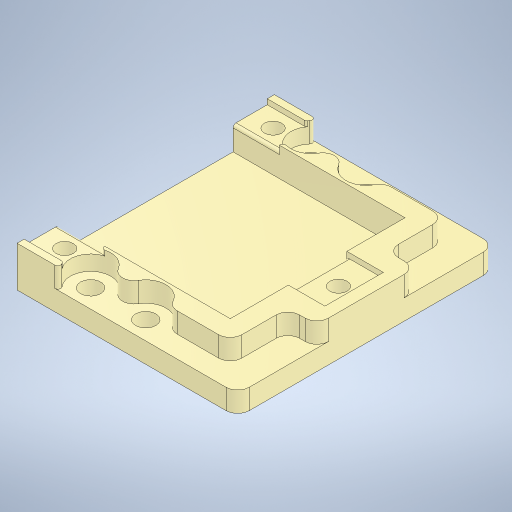
# Autodesk Inventor part: Servo Support
Saved by Autodesk Inventor 2023.4 (Build 274418000, 418)
## iProperties
Created: 2024-01-22
Part Number: Servo Support
Material: Nylon 6/6
Document SubType Name: Modeling
Designer: Nathan Cai
Density: 1.13 g/cm^3
Appearance: Nylon 6
Mass: 6.26234 g
Surface Area: 50.527 cm^2
Volume: 5.5419 cm^3
Author: Nathan Cai
Autodesk Inventor part; units mm, degrees
ref_plane "YZ Plane" through (0, 0, 0) normal (1, 0, 0) x (0, 1, 0)
ref_plane "XZ Plane" through (0, 0, 0) normal (0, 1, 0) x (-1, 0, 0)
ref_plane "XY Plane" through (0, 0, 0) normal (0, 0, 1) x (1, 0, 0)
sketch "Sketch8" plane through (0, 0, 0) normal (0, 1, 0) x (-1, 0, 0)
  line L0 (-14.8, 15) -> (14.8, 15)
  line L1 (14.8, 15) -> (14.8, -15)
  line L2 (14.8, -15) -> (-14.8, -15)
  line L3 (-14.8, -15) -> (-14.8, 15)
  line L4 (-14.8, 15) -> (14.8, -15) construction
  line L5 (14.8, 15) -> (-14.8, -15) construction
  line L6 (14.8, 0) -> (-14.8, 0) construction
  line L7 (14.8, 21) -> (6.8, 21)
  line L8 (6.8, 21) -> (6.8, -21)
  line L9 (6.8, -21) -> (14.8, -21)
  line L10 (14.8, -21) -> (14.8, 21)
  line L11 (14.8, 21) -> (6.8, -21) construction
  line L12 (6.8, 21) -> (14.8, -21) construction
  line L13 (10.8, 21) -> (10.8, -21) construction
  circle A0 centre (10.8, 18) radius 1.5
  circle A1 centre (10.8, -18) radius 1.5
  line L14 (-21.2, 5.05) -> (-14.8, 5.05)
  line L15 (-14.8, 5.05) -> (-14.8, -5.05)
  line L16 (-14.8, -5.05) -> (-21.2, -5.05)
  line L17 (-21.2, -5.05) -> (-21.2, 5.05)
  line L18 (-21.2, 5.05) -> (-14.8, -5.05) construction
  line L19 (-14.8, 5.05) -> (-21.2, -5.05) construction
  circle A2 centre (-18.5, 0) radius 1.5
  line L20 (24.325, 14.4) -> (14.8, 14.4)
  line L21 (14.8, 14.4) -> (14.8, 2.4)
  line L22 (14.8, 2.4) -> (24.325, 2.4)
  line L23 (24.325, 2.4) -> (24.325, 14.4)
  line L24 (24.325, 14.4) -> (14.8, 2.4) construction
  line L25 (14.8, 14.4) -> (24.325, 2.4) construction
  line L26 (-23.3, 22.225) -> (14.8, 22.225)
  line L27 (14.8, 22.225) -> (14.8, -22.225)
  line L28 (14.8, -22.225) -> (-23.3, -22.225)
  line L29 (-23.3, -22.225) -> (-23.3, 22.225)
  line L30 (-23.3, 22.225) -> (14.8, -22.225) construction
  line L31 (14.8, 22.225) -> (-23.3, -22.225) construction
  point P0 (0, 0)
  point P1 (10.8, 0)
  point P2 (-18, 0)
  point P3 (19.5625, 8.4)
  point P4 (-4.25, 0)
  point P5 (14.8, 21)
  point P6 (-14.8, 5.05)
  point P7 (6.8, -15)
  point P8 (14.8, 15)
  point P9 (6.8, 15)
  dimension "d120" = 29.6
  dimension "d121" = 30
  dimension "d122" = 8
  dimension "d123" = 42
  dimension "d124" = 3
  dimension "d126" = 36
  dimension "d127" = 10.1
  dimension "d128" = 36
  dimension "d129" = 3
  dimension "d130" = 29.3
  dimension "d131" = 9.6
  dimension "d132" = 12
  dimension "d133" = 9.525
  dimension "d134" = 44.45
  dimension "d135" = 38.1
  constraints: 64 end point, 14 midpoint, 10 parallel, 9 point on line, 5 horizontal, 5 perpendicular, 3 centre point, 1 symmetric about line, 1 other
  measures "d120" distance of L1.end L2.end
  measures "d121" distance of L0.end L1.end
  measures "d122" distance of L9.end L8.end
  measures "d123" distance of L8.end L7.end
  measures "d124" diameter of A0
  measures "d126" distance between parallel lines of L1 L17
  measures "d127" distance between parallel lines of L14 L16
  measures "d128" distance of A1.centre A0.centre
  measures "d129" diameter of A2
  measures "d130" distance from line of L13 A2.centre
  measures "d131" vertical distance of A0.centre point (19.563, 8.4)
  measures "d132" distance between parallel lines of L22 L20
  measures "d133" distance between parallel lines of L21 L23
  measures "d134" distance between parallel lines of L28 L26
  measures "d135" distance between parallel lines of L27 L29
extrude "Extrusion12" add sketch "Sketch8" against normal blind 7 contours L3 L14 L17 L16 L2 L8 L9 L27 L28 L29 L26 L7 L0 | L0 L8 L2 L3 | L8 L7 L10 L0 | L0 L1 L2 L8 | L3 L16 L17 L14 | L2 L10 L9 L8 | A0 | A1 | A2
extrude "Extrusion13" cut sketch "Sketch8" against normal blind 5 contours L0 L8 L2 L3 | L0 L1 L2 L8
extrude "Extrusion14" cut sketch "Sketch8" against normal blind 0.9 contours L8 L7 L10 L0 | L3 L16 L17 L14 | L2 L10 L9 L8 | A0 | A1 | A2
extrude "Extrusion15" cut sketch "Sketch8" against normal through all contours A0 | A1 | A2
shell "Shell1" thickness 3.5 removed faces 5 at (10.4333, 0, -19.4083) at (-2.1, -2.3333, 22.225) at (-14.8, -6.3333, -5) at (23.3, -2.3333, 7.4083) at (10.6, -2.3333, -22.225)
fillet "Fillet7" radius 0.5 5 edges at (-10.8, -0.9, -15) (14.8, -0.9, 0) (14.8, -0.9, 4.2065) (14.8, -0.9, -4.2065) (-10.8, -0.9, 15)
fillet "Fillet8" radius 2 12 edges at (-3.3, -1.75, 18.5) (18.3, -1.75, 18.5) (18.3, -1.75, 8.55) (18.3, -1.75, -8.55) (18.3, -1.75, -18.5) (-3.3, -1.75, -18.5) (23.3, -1.75, 8.55) (23.3, -1.75, -8.55) (-3.3, -1.75, 22.225) (-3.3, -1.75, -22.225) (23.3, -5.25, 22.225) (23.3, -5.25, -22.225)
sketch "Sketch9" plane through (0, 0, 0) normal (0, 1, 0) x (1, 0, 0)
  arc A0 (-3.2953, 20.3625) -> (-1.3, 18.5) centre (-1.3, 20.5) ccw projected
  line L0 (-1.3, 18.5) -> (16.3, 18.5) projected
  arc A1 (18.3, 16.5) -> (16.3, 18.5) centre (16.3, 16.5) ccw projected
  line L1 (18.3, 16.5) -> (18.3, 10.55) projected
  arc A2 (18.3, 10.55) -> (20.3, 8.55) centre (20.3, 10.55) ccw projected
  line L2 (20.3, 8.55) -> (21.3, 8.55) projected
  line L3 (23.3, 20.225) -> (23.3, 6.55) projected
  line L4 (-5.2905, 22.225) -> (21.3, 22.225) projected
  arc A3 (-3.2953, 20.3625) -> (-5.2905, 22.225) centre (-5.2905, 20.225) ccw projected
  arc A4 (20.3, -8.55) -> (18.3, -10.55) centre (20.3, -10.55) ccw projected
  line L5 (18.3, -10.55) -> (18.3, -16.5) projected
  arc A5 (16.3, -18.5) -> (18.3, -16.5) centre (16.3, -16.5) ccw projected
  line L6 (16.3, -18.5) -> (-1.3, -18.5) projected
  arc A6 (-1.3, -18.5) -> (-3.2953, -20.3625) centre (-1.3, -20.5) ccw projected
  arc A7 (-5.2905, -22.225) -> (-3.2953, -20.3625) centre (-5.2905, -20.225) ccw projected
  line L7 (21.3, -22.225) -> (-5.2905, -22.225) projected
  line L8 (23.3, 20.225) -> (23.3, 6.55) projected
  line L9 (21.3, -8.55) -> (20.3, -8.55) projected
  line L10 (-5.2905, 22.225) -> (23.3, 22.225) projected
  line L11 (23.3, -22.225) -> (-5.2905, -22.225) projected
  line L12 (23.3, 22.225) -> (9.0125, 22.225)
  line L13 (9.0125, 22.225) -> (9.0125, -22.225)
  line L14 (9.0125, -22.225) -> (23.3, -22.225)
  line L15 (23.3, -22.225) -> (23.3, 22.225)
  line L16 (23.3, 22.225) -> (23.3, 6.55) projected
  line L17 (23.3, 19.05) -> (-14.8, 19.05) construction
  line L18 (-14.8, 22.225) -> (-14.8, 21) projected
  line L19 (-14.8, -15) -> (-14.8, 15) projected
  line L20 (-14.8, 0) -> (23.3, 0) construction
  circle A8 centre (4.25, 19.05) radius 1.7526
  circle A9 centre (-5.275, 19.05) radius 1.7526
  circle A10 centre (4.25, -19.05) radius 1.7526
  circle A11 centre (-5.275, -19.05) radius 1.7526
  circle A12 centre (4.25, 19.05) radius 3.5
  circle A13 centre (-5.275, 19.05) radius 3.5
  circle A14 centre (4.25, -19.05) radius 3.5
  circle A15 centre (-5.275, -19.05) radius 3.5
  arc A16 (-3.2953, 20.3625) -> (-1.3, 18.5) centre (-1.3, 20.5) ccw projected
  line L21 (-1.3, 18.5) -> (16.3, 18.5) projected
  arc A17 (18.3, 16.5) -> (16.3, 18.5) centre (16.3, 16.5) ccw projected
  line L22 (18.3, 16.5) -> (18.3, 10.55) projected
  arc A18 (18.3, 10.55) -> (20.3, 8.55) centre (20.3, 10.55) ccw projected
  line L23 (20.3, 8.55) -> (21.3, 8.55) projected
  line L24 (-5.2905, 22.225) -> (21.3, 22.225) projected
  arc A19 (-3.2953, 20.3625) -> (-5.2905, 22.225) centre (-5.2905, 20.225) ccw projected
  line L25 (21.3, -8.55) -> (20.3, -8.55) projected
  arc A20 (20.3, -8.55) -> (18.3, -10.55) centre (20.3, -10.55) ccw projected
  line L26 (18.3, -10.55) -> (18.3, -16.5) projected
  arc A21 (16.3, -18.5) -> (18.3, -16.5) centre (16.3, -16.5) ccw projected
  line L27 (16.3, -18.5) -> (-1.3, -18.5) projected
  arc A22 (-1.3, -18.5) -> (-3.2953, -20.3625) centre (-1.3, -20.5) ccw projected
  arc A23 (-5.2905, -22.225) -> (-3.2953, -20.3625) centre (-5.2905, -20.225) ccw projected
  line L28 (21.3, -22.225) -> (-5.2905, -22.225) projected
  arc A24 (21.3, -8.55) -> (23.3, -6.55) centre (21.3, -6.55) ccw projected
  arc A25 (23.3, 6.55) -> (21.3, 8.55) centre (21.3, 6.55) ccw projected
  line L29 (23.3, -6.55) -> (23.3, -20.225) projected
  line L30 (23.3, -6.55) -> (23.3, -20.225) projected
  arc A26 (21.3, -8.55) -> (23.3, -6.55) centre (21.3, -6.55) ccw projected
  arc A27 (23.3, 6.55) -> (21.3, 8.55) centre (21.3, 6.55) ccw projected
  arc A28 (23.3, 20.225) -> (21.3, 22.225) centre (21.3, 20.225) ccw projected
  arc A29 (21.3, -22.225) -> (23.3, -20.225) centre (21.3, -20.225) ccw projected
  arc A30 (23.3, 20.225) -> (21.3, 22.225) centre (21.3, 20.225) ccw projected
  arc A31 (21.3, -22.225) -> (23.3, -20.225) centre (21.3, -20.225) ccw projected
  point P0 (0, 0)
  point P1 (9.0125, -18.5)
  point P2 (9.0125, 22.225)
  point P3 (9.0125, 18.5)
  point P4 (9.0125, 18.5)
  point P5 (9.0125, 22.225)
  point P6 (29.65, 22.225)
  point P7 (9.0125, -18.5)
  point P8 (29.65, -22.225)
  point P9 (9.0125, -22.225)
  point P10 (2.5859, 18.5)
  point P11 (5.9141, 18.5)
  point P12 (-0.5891, 18.5)
  point P13 (2.7391, 18.5)
  point P14 (2.5859, -18.5)
  point P15 (5.9141, -18.5)
  point P16 (-0.5891, -18.5)
  point P17 (2.7391, -18.5)
  point P18 (-3.2931, 20.3338)
  point P19 (-3.2931, -20.3338)
  dimension "d147" = 14.2875
  dimension "d148" = 19.05
  dimension "d149" = 3.5052
  dimension "d150" = 4.7625
  dimension "d153" = 9.525
  dimension "d161" = 7
  dimension "d164" = 9.525
  constraints: 12 end point, 8 centre point, 4 symmetric about line, 3 horizontal, 3 midpoint, 3 parallel, 3 point on line, 1 coincident, 1 perpendicular, 8 other
  measures "d147" distance between parallel lines of L15 L13
  measures "d148" distance between parallel lines of L20 L17
  measures "d149" diameter of A8
  measures "d150" distance from line of L13 A8.centre
  measures "d153" distance of A8.centre A9.centre
  measures "d161" diameter of A12
  measures "d164" distance of A12.centre A13.centre
extrude "Extrusion16" cut sketch "Sketch9" against normal blind 10 contours A8 L0 | L0 A8 | A10 L6 | L6 A10 | A9 | A11
extrude "Extrusion17" cut sketch "Sketch9" against normal up to surface (3.5 mm away) contours A3 L4 A13 A0 | A0 A13 L4 A3 | A12 L4 L0 A8 | L0 A8 A12 | A12 L4 | A8 L0 | L0 A8 | A14 L7 L6 A10 | L6 A10 A14 | A10 L6 | L6 A10 | A14 L7 | A15 L7 A7 A6 | A6 A7 L7 A15 | A9 | A11
fillet "Fillet10" radius 2 6 edges at (0.7935, -1.75, -18.5) (7.7065, -1.75, -18.5) (7.7065, -1.75, 18.5) (0.7935, -1.75, 18.5) (-1.8087, -1.75, -18.5658) (-1.8087, -1.75, 18.5658)
thicken "Thicken3" operation add thickness 0.1 both sides no extend neighbours yes toward (0, 0, -1) faces at (7.6, -2.1333, -15) (14.8, -3.8, 1.6833) (7.6, -2.1333, 15)
fillet "Fillet11" radius 0.5 6 edges at (-6.7479, -1.75, -22.225) (-8.1815, -0.45, -21) (-6.8, -0.45, -15.8997) (-6.8, -0.45, 15.8997) (-8.1815, -0.45, 21) (-6.7479, -1.75, 22.225)
body "Solid3"
